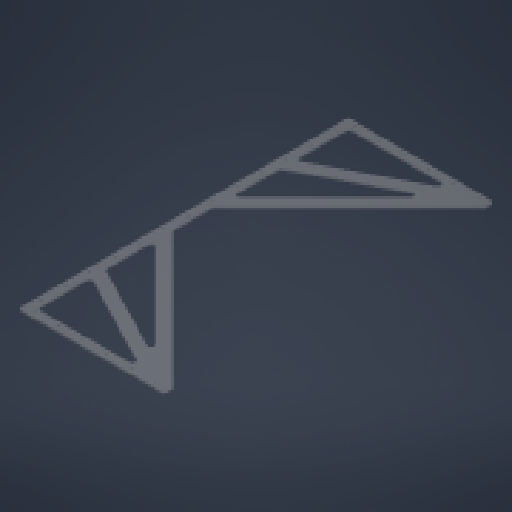
# Autodesk Inventor part: TOP_INTAKE_LEXAN
Saved by Autodesk Inventor 2026.2 (Build 302298010, 298A)
## iProperties
Created: 2026-04-02
Part Number: TOP_INTAKE_LEXAN
Material: Polycarbonate, PC 1000, Clear
Document SubType Name: Sheet Metal
Designer: 4aida
Density: 1.20131 g/cm^3
Sheet Metal Rule: Default_mm
Appearance: Lexan (Clear)
Author: 4aida
Autodesk Inventor part; units mm, degrees
ref_plane "YZ Plane" through (0, 0, 0) normal (1, 0, 0) x (0, 1, 0)
ref_plane "XZ Plane" through (0, 0, 0) normal (0, 1, 0) x (-1, 0, 0)
ref_plane "XY Plane" through (0, 0, 0) normal (0, 0, 1) x (1, 0, 0)
sketch "Sketch1" plane through (0, 0, 0) normal (0, 1, 0) x (-1, 0, 0)
  line L0 (-150.8125, -342.392) -> (150.8125, -342.392)
  line L1 (150.8125, -342.392) -> (150.8125, 342.392)
  line L2 (150.8125, 342.392) -> (-150.8125, 342.392)
  line L3 (-150.8125, 342.392) -> (-150.8125, -342.392)
  line L4 (-150.8125, -342.392) -> (150.8125, 342.392) construction
  line L5 (150.8125, -342.392) -> (-150.8125, 342.392) construction
  line L6 (131.7625, -323.342) -> (131.7625, 323.342)
  line L7 (131.7625, 323.342) -> (-150.8125, 323.342)
  line L8 (131.7625, -323.342) -> (-150.8125, -323.342)
  line L9 (-150.8125, -323.342) -> (131.7625, -40.767)
  line L10 (131.7625, -76.688) -> (-114.8915, -323.342)
  line L11 (-85.759, -294.2096) -> (131.7625, -180.975)
  line L12 (131.7625, -209.6105) -> (-86.7136, -323.342)
  line L13 (131.7625, -195.2928) -> (-150.8125, -342.392) construction
  line L14 (131.7625, 0) -> (76.1788, 0)
  line L15 (-150.8125, 323.342) -> (131.7625, 40.767)
  line L16 (131.7625, 76.688) -> (-114.8915, 323.342)
  line L17 (-85.759, 294.2096) -> (131.7625, 180.975)
  line L18 (131.7625, 209.6105) -> (-86.7136, 323.342)
  point P0 (0, 0)
  point P1 (131.7625, 195.2928)
  point P2 (131.7625, 40.767)
  dimension "d0" = 19.05
  dimension "d1" = 19.05
  dimension "d2" = 19.05
  dimension "d4" = 282.575
  dimension "d5" = 646.684
  dimension "d6" = 25.4
  dimension "d7" = 45
  dimension "d9" = 25.4
  dimension "d10" = 12.7
  dimension "d11" = 17.5
  measures "d0" distance between parallel lines of L1 L6
  measures "d1" distance between parallel lines of L7 L2
  measures "d2" distance between parallel lines of L0 L8
  measures "d4" distance between parallel lines of L3 L6
  measures "d5" distance of L6.start L6.end
  measures "d6" distance between parallel lines of L10 L9
  measures "d7" angle of L8 L10
  measures "d9" distance between parallel lines of L12 L11
  measures "d10" distance between parallel lines of L13 L11
  measures "d11" angle of L11 L10
extrude "Plate1" add sketch "Sketch1" along normal blind 3.175 contours L3 L8 L6 L7 L2 L1 L0 | L9 L6 L10 L8 | L7 L16 L6 L15 | L10 L11 L6 L12 L8 | L7 L18 L6 L17 L16
fillet "Corner Round1" radius 6.35 20 edges at (-150.8125, 1.5875, 342.392) (150.8125, 1.5875, 342.392) (150.8125, 1.5875, 323.342) (86.7136, 1.5875, 323.342) (85.759, 1.5875, 294.2096) (-131.7625, 1.5875, 209.6105) (-131.7625, 1.5875, 323.342) (-131.7625, 1.5875, 180.975) (-131.7625, 1.5875, 76.688) (-131.7625, 1.5875, 40.767) (-131.7625, 1.5875, -40.767) (-131.7625, 1.5875, -76.688) (-131.7625, 1.5875, -180.975) (-131.7625, 1.5875, -209.6105) (85.759, 1.5875, -294.2096) (150.8125, 1.5875, -323.342) (150.8125, 1.5875, -342.392) (-150.8125, 1.5875, -342.392) (86.7136, 1.5875, -323.342) (-131.7625, 1.5875, -323.342)
sketch "Sketch2" plane through (0, 0, 0) normal (0, -1, 0) x (1, 0, 0)
  line L0 (-144.4625, 342.392) -> (144.4625, 342.392) projected
  line L1 (150.8125, 336.042) -> (150.8125, 325.9723) projected
  line L2 (-131.7625, 38.1367) -> (-131.7625, -38.1367) projected
  point P0 (0, 0)
  point P1 (125.4125, 332.867)
  point P2 (74.6125, 332.867)
  point P3 (23.8125, 332.867)
  point P4 (-26.9875, 332.867)
  point P5 (-77.7875, 332.867)
  point P6 (-128.5875, 332.867)
  point P7 (-141.2875, 0)
  point P8 (-131.7625, 0)
  point P9 (-141.2875, 50.8)
  point P10 (-141.2875, 101.6)
  point P11 (-141.2875, 152.4)
  point P12 (-141.2875, 203.2)
  point P13 (-141.2875, 254)
  point P14 (-141.2875, 304.8)
  dimension "d14" = 9.525
  dimension "d15" = 25.4
  dimension "d18" = 50.8
  dimension "d23" = 9.525
  dimension "d26" = 50.8
  constraints: 1 horizontal, 1 horizontal alignment, 1 midpoint, 1 vertical, 11 other
  measures "d14" distance from line of L0 point (125.413, 332.867)
  measures "d15" distance from line of L1 point (125.413, 332.867)
  measures "d18" distance of point (125.413, 332.867) point (74.613, 332.867)
  measures "d23" distance from line of L2 point (-141.288, 0)
  measures "d26" distance of point (-141.288, 0) point (-141.288, 50.8)
hole "Hole1" at (125.4125, 0, 332.867) at (74.6125, 0, 332.867) at (23.8125, 0, 332.867) at (-26.9875, 0, 332.867) at (-77.7875, 0, 332.867) at (-128.5875, 0, 332.867) at (-141.2875, 0, 0) at (-141.2875, 0, 50.8) at (-141.2875, 0, 101.6) at (-141.2875, 0, 152.4) at (-141.2875, 0, 203.2) at (-141.2875, 0, 254) at (-141.2875, 0, 304.8) direction (0, 1, 0) diameter 5.105 end through all clearance for "Flat Head Machine Screw (82)" size "#10" standard "Ansi Unified Screw Threads"
mirror "Mirror1" about plane through (0, 0, 0) normal (0, 0, 1) of "Hole1"
equation "\"d1\" = d0"
equation "\"d2\" = d0"
equation "\"d9\" = d6"
equation "\"d10\" = 0.5 * d9"
equation "\"d36\" = Thickness"
equation "\"d12\" = Thickness"
equation "\"BendRadius\" = Thickness"
equation "\"BendReliefWidth\" = Thickness"
equation "\"BendReliefDepth\" = 0.5 * Thickness"
equation "\"CornerReliefSize\" = 4 * Thickness"
equation "\"MinimumRemnant\" = 2 * Thickness"
equation "\"TransitionRadius\" = BendRadius"
equation "\"JacobiRadiusSize\" = BendRadius"
equation "\"GapSize\" = Thickness"
equation "\"Thickness\" = 3.175"
body "Solid1"
